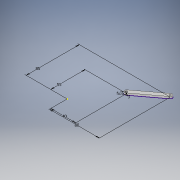
# Autodesk Inventor part: test
Saved by Autodesk Inventor 2019 (Build 230136000, 136)
## iProperties
Created: 2021-02-06
Part Number: test
Material: 一般
Document SubType Name: Modeling
Designer: wasd5
Density: 1 g/cm^3
Appearance: 預設
Author: wasd5
Autodesk Inventor part; units mm, degrees
ref_plane "YZ Plane" through (0, 0, 0) normal (1, 0, 0) x (0, 1, 0)
ref_plane "XZ Plane" through (0, 0, 0) normal (0, 1, 0) x (-1, 0, 0)
ref_plane "XY Plane" through (0, 0, 0) normal (0, 0, 1) x (1, 0, 0)
sketch "草圖3" plane through (0, 0, 0) normal (0, 1, 0) x (-1, 0, 0)
  line L0 (-37.6, -53.2) -> (-82.4, -86.8) construction
  line L1 (-38.2, -57.4) -> (-78.2, -87.4)
  line L2 (-81.8, -82.6) -> (-41.8, -52.6)
  arc A0 (-38.2, -57.4) -> (-41.8, -52.6) centre (-40, -55) ccw
  arc A1 (-81.8, -82.6) -> (-78.2, -87.4) centre (-80, -85) ccw
  circle A2 centre (-40, -55) radius 1.5
  circle A3 centre (-80, -85) radius 1.5
  point P0 (0, 0)
  point P1 (-60, -70)
  dimension "x1" = 40
  dimension "y1" = 55
  dimension "x2" = 80
  dimension "y2" = 85
  dimension "hole" = 3
  dimension "d14" = 6
  constraints: 8 end point, 6 point on circle, 4 centre point, 4 tangent, 2 coincident, 2 point on line, 1 equal radius, 1 midpoint, 1 parallel
  measures "x1" horizontal distance of point (0, 0) A0.centre
  measures "y1" vertical distance of point (0, 0) A0.centre
  measures "x2" horizontal distance of point (0, 0) A1.centre
  measures "y2" vertical distance of point (0, 0) A1.centre
  measures "hole" diameter of A2
  measures "d14" distance between parallel lines of L1 L2
extrude "擠出3" add sketch "草圖3" along normal blind 3
equation "\"d14\" = 2 * hole"
